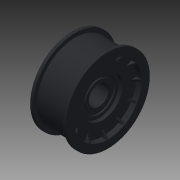
# Autodesk Inventor part: TPBSN38-15
Saved by Autodesk Inventor 2014 SP2 (Build 180246200, 246)
## iProperties
Created: 2018-08-04
Part Number: TPBSN38-15
Material: Generic
Catalog Web Link: www.cadenas.de
Description: TPBSN,TPCFN-Idlers
Vendor: MISUMI
Document SubType Name: Modeling
Designer: psadmin
Manufacturer: MISUMI
Mass: 14.3884 g
Surface Area: 66.5133 cm^2
Volume: 14.3884 cm^3
Density: 1 g/cm^3
Appearance: PSOLRGB-61-63-66
Category: PARTsolutions
Company: MISUMI
Title: TPBSN38-15
Author: Cadenas PARTsolutions
Comments: Idlers
PSOL_IDENT_0: {$CADENAS_DATA\23d-libs\misumi\metric\51_timing_pulleys\tpbsn.prj},167 {VTYP=3D},{NB=TPBSN38-15},{LI
PSOL_IDENT_1: NA=TPBSN38-15},{NN=TPBSN,TPCFN},{DATE=30.03.2018 07:26:35},{GEOMDATE=19.03.2015 00:00:00},{VERSION=}
PSOL_IDENT_2: ,{LINEID=10},{WBVAR=TS},{WBNUMERIC=}  {NB=TPBSN38-15},{LINA=TPBSN38-15},{KT=DUMMY},{PN=TPBSN38-15},{
PSOL_IDENT_3: TS=TPBSN},{MAT=Glass Reinforced Nylon},{OT=80 degree or Less},{TYPE=TPBSN},{D=38},{W=15},{W01=15},{W
PSOL_IDENT_4: 1=0},{W11=18},{F=42},{F1=42},{L=18},{L1=18},{S=4.5},{BN=6200ZZ},{DD=10},{B=9},{AID=WS010S},{TSA='TPB
PSOL_IDENT_5: SN','Flanged Idler','TPCFN','Flat Idler'}
NN: TPBSN,TPCFN
NT: Idlers
NB: TPBSN38-15
NBSYN: $PN.
LINA: TPBSN38-15
PN: TPBSN38-15
TS: Flanged Idler
MAT: Glass Reinforced Nylon
OT: 80 degree or Less
D: 38
W: 15
W1: 0
F: 42
L: 18
S: 4.5
BN: 6200ZZ
DD: 10
B: 9
AID: WS010S
SUPPLIER: MISUMI
ARTICLENO: TPBSN38-15
BOMINFO: TPBSN38-15
CREATOR: CADENAS GmbH
Autodesk Inventor part; units mm, degrees
ref_plane "YZ Plane" through (0, 0, 0) normal (1, 0, 0) x (0, 1, 0)
ref_plane "XZ Plane" through (0, 0, 0) normal (0, 1, 0) x (-1, 0, 0)
ref_plane "XY Plane" through (0, 0, 0) normal (0, 0, 1) x (1, 0, 0)
sketch "Sketch_1" plane through (0, 0, 0) normal (0, 0, 1) x (1, 0, 0)
  line L0 (18, 0) -> (0, 0)
  line L1 (0, 17) -> (2.7, 17)
  line L2 (2.7, 17) -> (2.7, 10)
  line L3 (2.7, 10) -> (4.5, 10)
  line L4 (4.5, 10) -> (4.5, 8.3333)
  line L5 (4.5, 8.3333) -> (5.25, 8.3333)
  line L6 (5.25, 8.3333) -> (5.25, 6.6667)
  line L7 (5.25, 6.6667) -> (4.5, 6.6667)
  line L8 (4.5, 6.6667) -> (4.5, 5)
  line L9 (4.5, 5) -> (13.5, 5)
  line L10 (13.5, 5) -> (13.5, 6.6667)
  line L11 (13.5, 6.6667) -> (12.75, 6.6667)
  line L12 (12.75, 6.6667) -> (12.75, 8.3333)
  line L13 (12.75, 8.3333) -> (13.5, 8.3333)
  line L14 (13.5, 8.3333) -> (13.5, 10)
  line L15 (13.5, 10) -> (15.3, 10)
  line L16 (15.3, 10) -> (15.3, 17)
  line L17 (15.3, 17) -> (18, 17)
  line L18 (18, 17) -> (18, 21)
  line L19 (18, 21) -> (16.5, 21)
  line L20 (16.5, 21) -> (16.5, 19)
  line L21 (16.5, 19) -> (1.5, 19)
  line L22 (1.5, 19) -> (1.5, 21)
  line L23 (1.5, 21) -> (0, 21)
  line L24 (0, 21) -> (0, 17)
  constraints: 50 end point
revolve "Revolution1" add sketch "Sketch_1" angle 360 about axis through (18, 0, 0) along (1, 0, 0)
sketch "Sketch_3" plane through (2.7, 0, 0) normal (1, 0, 0) x (0, 0, -1)
  line L0 (0.5, 14.2) -> (-0.5, 14.2)
  line L1 (-0.5, 14.2) -> (-0.5, 18)
  line L2 (-0.5, 18) -> (0.5, 18)
  line L3 (0.5, 18) -> (0.5, 14.2)
  line L4 (0.5, 14.2) -> (-0.5, 14.2)
  constraints: 10 end point
revolve "Revolution2" add sketch "Sketch_3" angle 40 about axis through (2.7, 14.2, -0.5) along (0, 0, 1)
pattern_circular "Circular Pattern1" count 12 over 360 about axis through (2.7, 0, 0) along (1, 0, 0) of "Revolution2"
sketch "Sketch_5" plane through (15.3, 0, 0) normal (1, 0, 0) x (0, 0, -1)
  line L0 (0.5, 14.2) -> (-0.5, 14.2)
  line L1 (-0.5, 14.2) -> (-0.5, 18)
  line L2 (-0.5, 18) -> (0.5, 18)
  line L3 (0.5, 18) -> (0.5, 14.2)
  line L4 (0.5, 14.2) -> (-0.5, 14.2)
  constraints: 10 end point
revolve "Revolution3" add sketch "Sketch_5" angle 40 about axis through (15.3, 14.2, -0.5) along (0, 0, -1)
pattern_circular "Circular Pattern2" count 12 over 360 about axis through (15.3, 0, 0) along (1, 0, 0) of "Revolution3"
body "Solid1"
